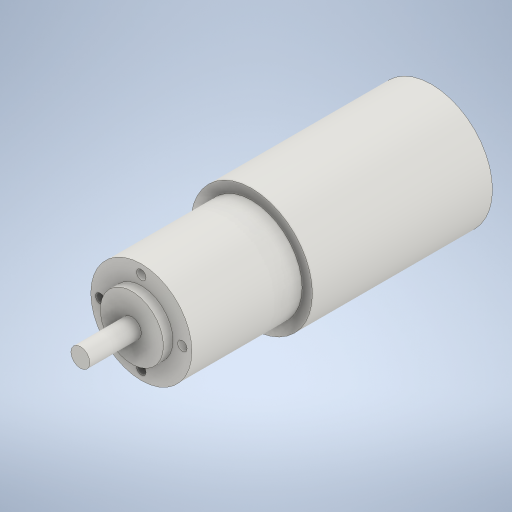
# Autodesk Inventor part: rs555vc5524
Saved by Autodesk Inventor 2024 (Build 280153000, 153)
## iProperties
Created: 2024-08-19
Part Number: rs555vc5524
Material: 一般
Document SubType Name: Modeling
Designer: yuki0520
Density: 1 g/cm^3
Appearance: 鋼
Author: yuki0520
Autodesk Inventor part; units mm, degrees
ref_plane "YZ Plane" through (0, 0, 0) normal (1, 0, 0) x (0, 1, 0)
ref_plane "XZ Plane" through (0, 0, 0) normal (0, 1, 0) x (-1, 0, 0)
ref_plane "XY Plane" through (0, 0, 0) normal (0, 0, 1) x (1, 0, 0)
sketch "スケッチ1" plane through (0, 0, 0) normal (0, 0, 1) x (1, 0, 0)
  circle A0 centre (0, 0) radius 19.25
  dimension "d0" = 38.5
  constraints: 1 centre point, 1 coincident
  measures "d0" diameter of A0
extrude "押し出し1" add sketch "スケッチ1" along normal blind 57
sketch "スケッチ2" plane through (0, 0, 57) normal (0, 0, 1) x (1, 0, 0)
  circle A0 centre (0, 0) radius 16
  dimension "d3" = 32
  constraints: 1 centre point, 1 coincident
  measures "d3" diameter of A0
extrude "押し出し2" add sketch "スケッチ2" along normal blind 34.9
sketch "スケッチ3" plane through (0, 0, 91.9) normal (0, 0, 1) x (1, 0, 0)
  circle A0 centre (0, 0) radius 3
  dimension "d6" = 6
  constraints: 1 centre point, 1 coincident
  measures "d6" diameter of A0
extrude "押し出し3" add sketch "スケッチ3" along normal blind 19.3
sketch "スケッチ4" plane through (0, 0, 91.9) normal (0, 0, 1) x (1, 0, 0)
  circle A0 centre (0, 0) radius 3 projected
  circle A1 centre (0, 0) radius 10
  dimension "d9" = 20
  constraints: 1 centre point, 1 coincident
  measures "d9" diameter of A1
extrude "押し出し4" add sketch "スケッチ4" along normal blind 3
sketch "スケッチ5" plane through (0, 0, 91.9) normal (0, 0, 1) x (1, 0, 0)
  circle A0 centre (0, 0) radius 3 projected
  circle A1 centre (0, 0) radius 13
  point P0 (0, 13)
  point P1 (-13, 0)
  point P2 (0, -13)
  point P3 (13, 0)
  dimension "d12" = 26
  dimension "d15" = 360
  constraints: 1 coincident, 1 vertical alignment, 7 other
hole "穴1" at (0, 13, 91.9) at (-13, 0, 91.9) at (0, -13, 91.9) at (13, 0, 91.9) direction (0, 0, -1) diameter 3 depth 4 tip angle 118
